Autodesk Fusion 360 part; units mm, degrees
(part 2 of 3)
sketch "Sketch24" plane through (0, 0, 3.2) normal (0, 0, 1) x (-1, 0, 0)
  line L0 (-121.4, -32.3) -> (-121.4, -38.2)
  line L1 (-121.4, -38.2) -> (-118.2, -38.2)
  line L2 (-118.2, -38.2) -> (-118.2, -48.2)
  line L3 (-118.2, -48.2) -> (-121.4, -48.2)
  line L4 (-121.4, -48.2) -> (-121.4, -54.1)
  line L5 (-121.4, -54.1) -> (-118.2, -54.1)
  line L6 (-118.2, -54.1) -> (-118.2, -64.1)
  line L7 (-118.2, -64.1) -> (-121.4, -64.1)
  line L8 (-121.4, -64.1) -> (-121.4, -70)
  line L9 (-121.4, -70) -> (-118.2, -70)
  line L10 (-118.2, -70) -> (-118.2, -80)
  line L11 (-118.2, -80) -> (-121.4, -80)
  line L12 (-121.4, -80) -> (-121.4, -86.4)
  line L13 (-121.4, -86.4) -> (-115, -86.4)
  line L14 (-115, -86.4) -> (-115, -83.2)
  line L15 (-115, -83.2) -> (-105, -83.2)
  line L16 (-105, -83.2) -> (-105, -86.4)
  line L17 (-105, -86.4) -> (-90.35, -86.4)
  line L18 (-90.35, -86.4) -> (-90.35, -83.2)
  line L19 (-90.35, -83.2) -> (-80.35, -83.2)
  line L20 (-80.35, -83.2) -> (-80.35, -86.4)
  line L21 (-80.35, -86.4) -> (-65.7, -86.4)
  line L22 (-65.7, -86.4) -> (-65.7, -83.2)
  line L23 (-65.7, -83.2) -> (-55.7, -83.2)
  line L24 (-55.7, -83.2) -> (-55.7, -86.4)
  line L25 (-55.7, -86.4) -> (-41.05, -86.4)
  line L26 (-41.05, -86.4) -> (-41.05, -83.2)
  line L27 (-41.05, -83.2) -> (-31.05, -83.2)
  line L28 (-31.05, -83.2) -> (-31.05, -86.4)
  line L29 (-31.05, -86.4) -> (-16.4, -86.4)
  line L30 (-16.4, -86.4) -> (-16.4, -83.2)
  line L31 (-16.4, -83.2) -> (-6.4, -83.2)
  line L32 (-6.4, -83.2) -> (-6.4, -86.4)
  line L33 (-6.4, -86.4) -> (0, -86.4)
  line L34 (0, -86.4) -> (0, -80)
  line L35 (0, -80) -> (-3.2, -80)
  line L36 (-3.2, -80) -> (-3.2, -70)
  line L37 (-3.2, -70) -> (0, -70)
  line L38 (0, -70) -> (0, -64.1)
  line L39 (0, -64.1) -> (-3.2, -64.1)
  line L40 (-3.2, -64.1) -> (-3.2, -54.1)
  line L41 (-3.2, -54.1) -> (0, -54.1)
  line L42 (0, -54.1) -> (0, -48.2)
  line L43 (0, -48.2) -> (-3.2, -48.2)
  line L44 (-3.2, -48.2) -> (-3.2, -38.2)
  line L45 (-3.2, -38.2) -> (0, -38.2)
  line L46 (0, -38.2) -> (0, -32.3)
  line L47 (0, -32.3) -> (-3.2, -32.3)
  line L48 (-3.2, -32.3) -> (-3.2, -22.3)
  line L49 (-3.2, -22.3) -> (0, -22.3)
  line L50 (0, -22.3) -> (0, -16.4)
  line L51 (0, -16.4) -> (-3.2, -16.4)
  line L52 (-3.2, -16.4) -> (-3.2, -6.4)
  line L53 (-3.2, -6.4) -> (0, -6.4)
  line L54 (0, -6.4) -> (0, 0)
  line L55 (0, 0) -> (-6.4, 0)
  line L56 (-6.4, 0) -> (-6.4, -3.2)
  line L57 (-6.4, -3.2) -> (-16.4, -3.2)
  line L58 (-16.4, -3.2) -> (-16.4, 0)
  line L59 (-16.4, 0) -> (-31.05, 0)
  line L60 (-31.05, 0) -> (-31.05, -3.2)
  line L61 (-31.05, -3.2) -> (-41.05, -3.2)
  line L62 (-41.05, -3.2) -> (-41.05, 0)
  line L63 (-41.05, 0) -> (-55.7, 0)
  line L64 (-55.7, 0) -> (-55.7, -3.2)
  line L65 (-55.7, -3.2) -> (-65.7, -3.2)
  line L66 (-65.7, -3.2) -> (-65.7, 0)
  line L67 (-65.7, 0) -> (-80.35, 0)
  line L68 (-80.35, 0) -> (-80.35, -3.2)
  line L69 (-80.35, -3.2) -> (-90.35, -3.2)
  line L70 (-90.35, -3.2) -> (-90.35, 0)
  line L71 (-90.35, 0) -> (-105, 0)
  line L72 (-105, 0) -> (-105, -3.2)
  line L73 (-105, -3.2) -> (-115, -3.2)
  line L74 (-115, -3.2) -> (-115, 0)
  line L75 (-115, 0) -> (-121.4, 0)
  line L76 (-121.4, 0) -> (-121.4, -6.4)
  line L77 (-121.4, -6.4) -> (-118.2, -6.4)
  line L78 (-118.2, -6.4) -> (-118.2, -16.4)
  line L79 (-118.2, -16.4) -> (-121.4, -16.4)
  line L80 (-121.4, -16.4) -> (-121.4, -22.3)
  line L81 (-121.4, -22.3) -> (-118.2, -22.3)
  line L82 (-118.2, -22.3) -> (-118.2, -32.3)
  line L83 (-118.2, -32.3) -> (-121.4, -32.3)
  line L84 (-8.2, -83.2) -> (-21.2, -83.2)
  line L85 (-23.2, -81.2) -> (-23.2, -80.2)
  line L86 (-21.2, -78.2) -> (-20.2, -78.2)
  line L87 (-18.2, -76.2) -> (-18.2, -35.2)
  line L88 (-20.2, -33.2) -> (-21.2, -33.2)
  line L89 (-23.2, -31.2) -> (-23.2, -5.2)
  line L90 (-21.2, -3.2) -> (-10.2, -3.2)
  line L91 (-8.2, -5.2) -> (-8.2, -26.2)
  line L92 (-6.2, -28.2) -> (-5.2, -28.2)
  line L93 (-3.2, -30.2) -> (-3.2, -81.2)
  line L94 (-5.2, -83.2) -> (-8.2, -83.2)
  arc A0 (-5.2, -83.2) -> (-3.2, -81.2) centre (-5.2, -81.2) ccw
  arc A1 (-23.2, -81.2) -> (-21.2, -83.2) centre (-21.2, -81.2) ccw
  arc A2 (-21.2, -78.2) -> (-23.2, -80.2) centre (-21.2, -80.2) ccw
  arc A3 (-20.2, -78.2) -> (-18.2, -76.2) centre (-20.2, -76.2) ccw
  arc A4 (-18.2, -35.2) -> (-20.2, -33.2) centre (-20.2, -35.2) ccw
  arc A5 (-23.2, -31.2) -> (-21.2, -33.2) centre (-21.2, -31.2) ccw
  arc A6 (-21.2, -3.2) -> (-23.2, -5.2) centre (-21.2, -5.2) ccw
  arc A7 (-8.2, -5.2) -> (-10.2, -3.2) centre (-10.2, -5.2) ccw
  arc A8 (-8.2, -26.2) -> (-6.2, -28.2) centre (-6.2, -26.2) ccw
  arc A9 (-3.2, -30.2) -> (-5.2, -28.2) centre (-5.2, -30.2) ccw
  line L95 (-23.2, -81.2) -> (-23.2, -70.2)
  line L96 (-25.2, -83.2) -> (-38.7, -83.2)
  line L97 (-40.7, -81.2) -> (-40.7, -80.2)
  line L98 (-42.7, -78.2) -> (-43.7, -78.2)
  line L99 (-45.7, -80.2) -> (-45.7, -81.2)
  line L100 (-47.7, -83.2) -> (-101.2, -83.2)
  line L101 (-25.2, -68.2) -> (-36.2, -68.2)
  line L102 (-38.2, -66.2) -> (-38.2, -65.2)
  line L103 (-40.2, -63.2) -> (-46.2, -63.2)
  line L104 (-48.2, -65.2) -> (-48.2, -66.2)
  line L105 (-50.2, -68.2) -> (-101.2, -68.2)
  line L106 (-103.2, -81.2) -> (-103.2, -70.2)
  arc A10 (-25.2, -83.2) -> (-23.2, -81.2) centre (-25.2, -81.2) ccw
  arc A11 (-23.2, -70.2) -> (-25.2, -68.2) centre (-25.2, -70.2) ccw
  arc A12 (-40.7, -81.2) -> (-38.7, -83.2) centre (-38.7, -81.2) ccw
  arc A13 (-40.7, -80.2) -> (-42.7, -78.2) centre (-42.7, -80.2) ccw
  arc A14 (-47.7, -83.2) -> (-45.7, -81.2) centre (-47.7, -81.2) ccw
  arc A15 (-43.7, -78.2) -> (-45.7, -80.2) centre (-43.7, -80.2) ccw
  arc A16 (-103.2, -81.2) -> (-101.2, -83.2) centre (-101.2, -81.2) ccw
  arc A17 (-101.2, -68.2) -> (-103.2, -70.2) centre (-101.2, -70.2) ccw
  arc A18 (-50.2, -68.2) -> (-48.2, -66.2) centre (-50.2, -66.2) ccw
  arc A19 (-46.2, -63.2) -> (-48.2, -65.2) centre (-46.2, -65.2) ccw
  arc A20 (-38.2, -65.2) -> (-40.2, -63.2) centre (-40.2, -65.2) ccw
  arc A21 (-38.2, -66.2) -> (-36.2, -68.2) centre (-36.2, -66.2) ccw
  line L107 (-18.2, -66.2) -> (-18.2, -55.2)
  line L108 (-20.2, -68.2) -> (-36.2, -68.2)
  line L109 (-38.2, -66.2) -> (-38.2, -65.2)
  line L110 (-40.2, -63.2) -> (-46.2, -63.2)
  line L111 (-48.2, -65.2) -> (-48.2, -66.2)
  line L112 (-50.2, -68.2) -> (-96.2, -68.2)
  line L113 (-98.2, -66.2) -> (-98.2, -55.2)
  arc A22 (-20.2, -68.2) -> (-18.2, -66.2) centre (-20.2, -66.2) ccw
  line L114 (-96.2, -53.2) -> (-55.2, -53.2)
  line L115 (-53.2, -51.2) -> (-53.2, -50.2)
  line L116 (-51.2, -48.2) -> (-35.2, -48.2)
  line L117 (-33.2, -50.2) -> (-33.2, -51.2)
  line L118 (-31.2, -53.2) -> (-20.2, -53.2)
  arc A23 (-38.2, -66.2) -> (-36.2, -68.2) centre (-36.2, -66.2) ccw
  arc A24 (-38.2, -65.2) -> (-40.2, -63.2) centre (-40.2, -65.2) ccw
  arc A25 (-46.2, -63.2) -> (-48.2, -65.2) centre (-46.2, -65.2) ccw
  arc A26 (-50.2, -68.2) -> (-48.2, -66.2) centre (-50.2, -66.2) ccw
  arc A27 (-98.2, -66.2) -> (-96.2, -68.2) centre (-96.2, -66.2) ccw
  arc A28 (-96.2, -53.2) -> (-98.2, -55.2) centre (-96.2, -55.2) ccw
  arc A29 (-55.2, -53.2) -> (-53.2, -51.2) centre (-55.2, -51.2) ccw
  arc A30 (-51.2, -48.2) -> (-53.2, -50.2) centre (-51.2, -50.2) ccw
  arc A31 (-33.2, -50.2) -> (-35.2, -48.2) centre (-35.2, -50.2) ccw
  arc A32 (-33.2, -51.2) -> (-31.2, -53.2) centre (-31.2, -51.2) ccw
  arc A33 (-18.2, -55.2) -> (-20.2, -53.2) centre (-20.2, -55.2) ccw
  line L119 (-18.2, -51.2) -> (-18.2, -38.2)
  line L120 (-20.2, -53.2) -> (-31.2, -53.2)
  line L121 (-33.2, -51.2) -> (-33.2, -50.2)
  line L122 (-35.2, -48.2) -> (-51.2, -48.2)
  line L123 (-53.2, -50.2) -> (-53.2, -51.2)
  line L124 (-55.2, -53.2) -> (-96.2, -53.2)
  line L125 (-98.2, -51.2) -> (-98.2, -40.2)
  line L126 (-96.2, -38.2) -> (-60.2, -38.2)
  line L127 (-58.2, -36.2) -> (-58.2, -35.2)
  line L128 (-56.2, -33.2) -> (-20.2, -33.2)
  line L129 (-18.2, -35.2) -> (-18.2, -38.2)
  arc A34 (-20.2, -53.2) -> (-18.2, -51.2) centre (-20.2, -51.2) ccw
  arc A35 (-33.2, -51.2) -> (-31.2, -53.2) centre (-31.2, -51.2) ccw
  arc A36 (-33.2, -50.2) -> (-35.2, -48.2) centre (-35.2, -50.2) ccw
  arc A37 (-55.2, -53.2) -> (-53.2, -51.2) centre (-55.2, -51.2) ccw
  arc A38 (-51.2, -48.2) -> (-53.2, -50.2) centre (-51.2, -50.2) ccw
  arc A39 (-98.2, -51.2) -> (-96.2, -53.2) centre (-96.2, -51.2) ccw
  arc A40 (-96.2, -38.2) -> (-98.2, -40.2) centre (-96.2, -40.2) ccw
  arc A41 (-60.2, -38.2) -> (-58.2, -36.2) centre (-60.2, -36.2) ccw
  arc A42 (-56.2, -33.2) -> (-58.2, -35.2) centre (-56.2, -35.2) ccw
  line L130 (-23.2, -31.2) -> (-23.2, -20.2)
  line L131 (-23.2, -18.2) -> (-23.2, -5.2)
  arc A43 (-18.2, -35.2) -> (-20.2, -33.2) centre (-20.2, -35.2) ccw
  line L132 (-25.2, -33.2) -> (-56.2, -33.2)
  line L133 (-58.2, -35.2) -> (-58.2, -36.2)
  line L134 (-60.2, -38.2) -> (-101.2, -38.2)
  line L135 (-103.2, -36.2) -> (-103.2, -20.2)
  line L136 (-101.2, -18.2) -> (-100.2, -18.2)
  line L137 (-98.2, -20.2) -> (-98.2, -21.2)
  line L138 (-96.2, -23.2) -> (-90.2, -23.2)
  line L139 (-88.2, -21.2) -> (-88.2, -20.2)
  line L140 (-86.2, -18.2) -> (-25.2, -18.2)
  arc A44 (-25.2, -33.2) -> (-23.2, -31.2) centre (-25.2, -31.2) ccw
  arc A45 (-56.2, -33.2) -> (-58.2, -35.2) centre (-56.2, -35.2) ccw
  arc A46 (-60.2, -38.2) -> (-58.2, -36.2) centre (-60.2, -36.2) ccw
  arc A47 (-103.2, -36.2) -> (-101.2, -38.2) centre (-101.2, -36.2) ccw
  arc A48 (-101.2, -18.2) -> (-103.2, -20.2) centre (-101.2, -20.2) ccw
  arc A49 (-98.2, -20.2) -> (-100.2, -18.2) centre (-100.2, -20.2) ccw
  arc A50 (-98.2, -21.2) -> (-96.2, -23.2) centre (-96.2, -21.2) ccw
  arc A51 (-90.2, -23.2) -> (-88.2, -21.2) centre (-90.2, -21.2) ccw
  arc A52 (-86.2, -18.2) -> (-88.2, -20.2) centre (-86.2, -20.2) ccw
  arc A53 (-23.2, -20.2) -> (-25.2, -18.2) centre (-25.2, -20.2) ccw
  line L141 (-23.2, -16.2) -> (-23.2, -3.2)
  line L142 (-25.2, -18.2) -> (-86.2, -18.2)
  line L143 (-88.2, -20.2) -> (-88.2, -21.2)
  line L144 (-90.2, -23.2) -> (-96.2, -23.2)
  line L145 (-98.2, -21.2) -> (-98.2, -20.2)
  line L146 (-100.2, -18.2) -> (-101.2, -18.2)
  line L147 (-103.2, -16.2) -> (-103.2, -5.2)
  line L148 (-101.2, -3.2) -> (-97.7, -3.2)
  line L149 (-95.7, -5.2) -> (-95.7, -6.2)
  line L150 (-93.7, -8.2) -> (-92.7, -8.2)
  line L151 (-90.7, -6.2) -> (-90.7, -5.2)
  line L152 (-88.7, -3.2) -> (-25.2, -3.2)
  arc A54 (-23.2, -5.2) -> (-25.2, -3.2) centre (-25.2, -5.2) ccw
  arc A55 (-25.2, -18.2) -> (-23.2, -16.2) centre (-25.2, -16.2) ccw
  arc A56 (-86.2, -18.2) -> (-88.2, -20.2) centre (-86.2, -20.2) ccw
  arc A57 (-90.2, -23.2) -> (-88.2, -21.2) centre (-90.2, -21.2) ccw
  arc A58 (-98.2, -21.2) -> (-96.2, -23.2) centre (-96.2, -21.2) ccw
  arc A59 (-98.2, -20.2) -> (-100.2, -18.2) centre (-100.2, -20.2) ccw
  arc A60 (-103.2, -16.2) -> (-101.2, -18.2) centre (-101.2, -16.2) ccw
  arc A61 (-101.2, -3.2) -> (-103.2, -5.2) centre (-101.2, -5.2) ccw
  arc A62 (-95.7, -5.2) -> (-97.7, -3.2) centre (-97.7, -5.2) ccw
  arc A63 (-95.7, -6.2) -> (-93.7, -8.2) centre (-93.7, -6.2) ccw
  arc A64 (-92.7, -8.2) -> (-90.7, -6.2) centre (-92.7, -6.2) ccw
  arc A65 (-88.7, -3.2) -> (-90.7, -5.2) centre (-88.7, -5.2) ccw
  line L153 (-116.2, -3.2) -> (-105.2, -3.2)
  line L154 (-103.2, -5.2) -> (-103.2, -36.2)
  line L155 (-101.2, -38.2) -> (-100.2, -38.2)
  line L156 (-98.2, -40.2) -> (-98.2, -66.2)
  line L157 (-100.2, -68.2) -> (-101.2, -68.2)
  line L158 (-103.2, -70.2) -> (-103.2, -81.2)
  line L159 (-105.2, -83.2) -> (-116.2, -83.2)
  line L160 (-118.2, -81.2) -> (-118.2, -62.7)
  line L161 (-116.2, -60.7) -> (-115.2, -60.7)
  line L162 (-113.2, -58.7) -> (-113.2, -47.7)
  line L163 (-115.2, -45.7) -> (-116.2, -45.7)
  line L164 (-118.2, -43.7) -> (-118.2, -5.2)
  arc A66 (-103.2, -5.2) -> (-105.2, -3.2) centre (-105.2, -5.2) ccw
  arc A67 (-116.2, -3.2) -> (-118.2, -5.2) centre (-116.2, -5.2) ccw
  arc A68 (-118.2, -43.7) -> (-116.2, -45.7) centre (-116.2, -43.7) ccw
  arc A69 (-113.2, -47.7) -> (-115.2, -45.7) centre (-115.2, -47.7) ccw
  arc A70 (-115.2, -60.7) -> (-113.2, -58.7) centre (-115.2, -58.7) ccw
  arc A71 (-116.2, -60.7) -> (-118.2, -62.7) centre (-116.2, -62.7) ccw
  arc A72 (-118.2, -81.2) -> (-116.2, -83.2) centre (-116.2, -81.2) ccw
  arc A73 (-105.2, -83.2) -> (-103.2, -81.2) centre (-105.2, -81.2) ccw
  arc A74 (-101.2, -68.2) -> (-103.2, -70.2) centre (-101.2, -70.2) ccw
  arc A75 (-100.2, -68.2) -> (-98.2, -66.2) centre (-100.2, -66.2) ccw
  arc A76 (-98.2, -40.2) -> (-100.2, -38.2) centre (-100.2, -40.2) ccw
  arc A77 (-103.2, -36.2) -> (-101.2, -38.2) centre (-101.2, -36.2) ccw
  point P0 (-23.2, -83.2)
  point P1 (-3.2, -83.2)
  point P2 (-23.2, -78.2)
  point P3 (-18.2, -78.2)
  point P4 (-18.2, -33.2)
  point P5 (-23.2, -33.2)
  point P6 (-23.2, -3.2)
  point P7 (-8.2, -3.2)
  point P8 (-8.2, -28.2)
  point P9 (-3.2, -28.2)
  point P10 (-23.2, -83.2)
  point P11 (-23.2, -68.2)
  point P12 (-40.7, -83.2)
  point P13 (-40.7, -78.2)
  point P14 (-45.7, -78.2)
  point P15 (-45.7, -83.2)
  point P16 (-103.2, -83.2)
  point P17 (-38.2, -68.2)
  point P18 (-38.2, -63.2)
  point P19 (-48.2, -63.2)
  point P20 (-48.2, -68.2)
  point P21 (-103.2, -68.2)
  point P22 (-18.2, -68.2)
  point P23 (-18.2, -53.2)
  point P24 (-38.2, -68.2)
  point P25 (-38.2, -63.2)
  point P26 (-38.2, -63.2)
  point P27 (-48.2, -63.2)
  point P28 (-48.2, -68.2)
  point P29 (-48.2, -68.2)
  point P30 (-98.2, -68.2)
  point P31 (-98.2, -53.2)
  point P32 (-53.2, -53.2)
  point P33 (-53.2, -48.2)
  point P34 (-33.2, -48.2)
  point P35 (-33.2, -53.2)
  point P36 (-18.2, -53.2)
  point P37 (-33.2, -53.2)
  point P38 (-33.2, -48.2)
  point P39 (-33.2, -48.2)
  point P40 (-53.2, -48.2)
  point P41 (-53.2, -48.2)
  point P42 (-53.2, -53.2)
  point P43 (-53.2, -53.2)
  point P44 (-98.2, -53.2)
  point P45 (-98.2, -38.2)
  point P46 (-58.2, -38.2)
  point P47 (-58.2, -33.2)
  point P48 (-18.2, -33.2)
  point P49 (-23.2, -33.2)
  point P50 (-23.2, -3.2)
  point P51 (-23.2, -33.2)
  point P52 (-58.2, -33.2)
  point P53 (-58.2, -38.2)
  point P54 (-58.2, -38.2)
  point P55 (-103.2, -38.2)
  point P56 (-103.2, -18.2)
  point P57 (-98.2, -18.2)
  point P58 (-98.2, -23.2)
  point P59 (-88.2, -23.2)
  point P60 (-88.2, -18.2)
  point P61 (-23.2, -18.2)
  point P62 (-23.2, -18.2)
  point P63 (-88.2, -18.2)
  point P64 (-88.2, -18.2)
  point P65 (-88.2, -23.2)
  point P66 (-98.2, -23.2)
  point P67 (-98.2, -18.2)
  point P68 (-103.2, -18.2)
  point P69 (-103.2, -18.2)
  point P70 (-103.2, -3.2)
  point P71 (-95.7, -3.2)
  point P72 (-95.7, -8.2)
  point P73 (-90.7, -8.2)
  point P74 (-90.7, -3.2)
  point P75 (-118.2, -3.2)
  point P76 (-103.2, -3.2)
  point P77 (-103.2, -38.2)
  point P78 (-103.2, -38.2)
  point P79 (-98.2, -38.2)
  point P80 (-98.2, -38.2)
  point P81 (-98.2, -68.2)
  point P82 (-98.2, -68.2)
  point P83 (-103.2, -68.2)
  point P84 (-103.2, -68.2)
  point P85 (-103.2, -83.2)
  point P86 (-103.2, -83.2)
  point P87 (-118.2, -83.2)
  point P88 (-118.2, -60.7)
  point P89 (-113.2, -60.7)
  point P90 (-113.2, -45.7)
  point P91 (-118.2, -45.7)
  point P92 (-118.2, -3.2)
  dimension "d178" = 15
  dimension "d179" = 5
  dimension "d180" = 5
  dimension "d181" = 5
  dimension "d182" = 45
  dimension "d183" = 5
  dimension "d185" = 15
  dimension "d186" = 25
  dimension "d187" = 5
  dimension "d188" = 2
  dimension "d189" = 8.2
  dimension "d190" = 2
  dimension "d191" = 2
  dimension "d192" = 2
  dimension "d193" = 2
  dimension "d194" = 2
  dimension "d195" = 2
  dimension "d196" = 2
  dimension "d197" = 2
  dimension "d198" = 2
  dimension "d202" = 30
  dimension "d203" = 80
  dimension "d204" = 15
  dimension "d205" = 23.2
  dimension "d206" = 83.2
  dimension "d208" = 17.5
  dimension "d209" = 5
  dimension "d210" = 5
  dimension "d211" = 5
  dimension "d212" = 57.5
  dimension "d213" = 15
  dimension "d214" = 5
  dimension "d215" = 10
  dimension "d216" = 5
  dimension "d218" = 55
  dimension "d219" = 2
  dimension "d220" = 2
  dimension "d221" = 2
  dimension "d222" = 2
  dimension "d223" = 2
  dimension "d224" = 2
  dimension "d225" = 2
  dimension "d226" = 2
  dimension "d227" = 2
  dimension "d228" = 2
  dimension "d229" = 2
  dimension "d230" = 2
  dimension "d231" = 15
  dimension "d232" = 18.2
  dimension "d233" = 68.2
  dimension "d234" = 20
  dimension "d235" = 5
  dimension "d237" = 10
  dimension "d238" = 5
  dimension "d239" = 50
  dimension "d240" = 15
  dimension "d241" = 2
  dimension "d242" = 5
  dimension "d243" = 5
  dimension "d244" = 20
  dimension "d245" = 5
  dimension "d246" = 2
  dimension "d247" = 2
  dimension "d248" = 2
  dimension "d249" = 2
  dimension "d250" = 2
  dimension "d251" = 2
  dimension "d252" = 2
  dimension "d253" = 2
  dimension "d254" = 2
  dimension "d255" = 2
  dimension "d256" = 2
  dimension "d257" = 15
  dimension "d258" = 18.2
  dimension "d259" = 53.2
  dimension "d260" = 15
  dimension "d261" = 5
  dimension "d262" = 20
  dimension "d263" = 5
  dimension "d264" = 45
  dimension "d265" = 15
  dimension "d266" = 40
  dimension "d267" = 5
  dimension "d268" = 40
  dimension "d269" = 2
  dimension "d270" = 2
  dimension "d271" = 2
  dimension "d272" = 2
  dimension "d273" = 2
  dimension "d274" = 2
  dimension "d275" = 2
  dimension "d276" = 2
  dimension "d277" = 2
  dimension "d278" = 15
  dimension "d279" = 23.2
  dimension "d280" = 33.2
  dimension "d281" = 2
  dimension "d282" = 35
  dimension "d283" = 5
  dimension "d284" = 45
  dimension "d285" = 20
  dimension "d286" = 5
  dimension "d287" = 5
  dimension "d288" = 10
  dimension "d289" = 5
  dimension "d290" = 65
  dimension "d291" = 15
  dimension "d292" = 40
  dimension "d293" = 2
  dimension "d294" = 2
  dimension "d295" = 2
  dimension "d296" = 2
  dimension "d297" = 2
  dimension "d298" = 2
  dimension "d299" = 2
  dimension "d300" = 2
  dimension "d301" = 2
  dimension "d302" = 2
  dimension "d303" = 15
  dimension "d304" = 3.2
  dimension "d305" = 23.2
  dimension "d306" = 65
  dimension "d307" = 5
  dimension "d308" = 10
  dimension "d309" = 5
  dimension "d310" = 5
  dimension "d311" = 15
  dimension "d312" = 7.5
  dimension "d313" = 5
  dimension "d314" = 5
  dimension "d315" = 5
  dimension "d316" = 2
  dimension "d317" = 2
  dimension "d318" = 2
  dimension "d319" = 2
  dimension "d320" = 2
  dimension "d321" = 2
  dimension "d322" = 2
  dimension "d323" = 2
  dimension "d324" = 2
  dimension "d325" = 2
  dimension "d326" = 2
  dimension "d327" = 2
  dimension "d328" = 15
  dimension "d330" = 15
  dimension "d331" = 3.2
  dimension "d332" = 103.2
  dimension "d333" = 35
  dimension "d334" = 5
  dimension "d335" = 30
  dimension "d336" = 5
  dimension "d337" = 15
  dimension "d338" = 15
  dimension "d339" = 22.5
  dimension "d340" = 5
  dimension "d341" = 15
  dimension "d342" = 5
  dimension "d343" = 42.5
  dimension "d344" = 2
  dimension "d345" = 2
  dimension "d346" = 2
  dimension "d347" = 2
  dimension "d348" = 2
  dimension "d349" = 2
  dimension "d350" = 2
  dimension "d351" = 2
  dimension "d352" = 2
  dimension "d353" = 2
  dimension "d354" = 2
  dimension "d355" = 2
  constraint perpendicular L32 L84
  constraint perpendicular L84 L85
  constraint perpendicular L85 L86
  constraint perpendicular L86 L87
  constraint perpendicular L87 L88
  constraint perpendicular L88 L89
  constraint perpendicular L89 L90
  constraint perpendicular L57 L91
  constraint perpendicular L91 L92
  constraint perpendicular L35 L93
  constraint perpendicular L32 L94
  constraint tangent L93 A0
  constraint tangent L94 A0
  constraint coincident P10 L84
  constraint coincident P10 L85
  constraint tangent L84 A1
  constraint tangent L85 A1
  constraint coincident P2 L85
  constraint coincident P2 L86
  constraint tangent L85 A2
  constraint tangent L86 A2
  constraint coincident P3 L86
  constraint coincident P3 L87
  constraint tangent L86 A3
  constraint tangent L87 A3
  constraint coincident P48 L88
  constraint tangent L87 A4
  constraint tangent L88 A4
  constraint coincident P51 L88
  constraint coincident P51 L89
  constraint tangent L88 A5
  constraint tangent L89 A5
  constraint coincident P50 L89
  constraint coincident P50 L90
  constraint tangent L89 A6
  constraint tangent L90 A6
  constraint coincident P7 L90
  constraint coincident P7 L91
  constraint tangent L90 A7
  constraint tangent L91 A7
  constraint coincident P8 L91
  constraint coincident P8 L92
  constraint tangent L91 A8
  constraint tangent L92 A8
  constraint coincident P9 L92
  constraint coincident P9 L93
  constraint tangent L92 A9
  constraint tangent L93 A9
  constraint vertical L95
  constraint perpendicular L26 L96
  constraint perpendicular L27 L97
  constraint perpendicular L97 L98
  constraint perpendicular L98 L99
  constraint perpendicular L20 L100
  constraint perpendicular L95 L101
  constraint perpendicular L101 L102
  constraint perpendicular L102 L103
  constraint perpendicular L103 L104
  constraint perpendicular L104 L105
  constraint coincident P10 L95
  constraint coincident P10 L96
  constraint tangent L95 A10
  constraint tangent L96 A10
  constraint coincident P11 L95
  constraint coincident P11 L101
  constraint tangent L95 A11
  constraint tangent L101 A11
  constraint coincident P12 L96
  constraint coincident P12 L97
  constraint tangent L96 A12
  constraint tangent L97 A12
  constraint coincident P13 L97
  constraint coincident P13 L98
  constraint tangent L97 A13
  constraint tangent L98 A13
  constraint coincident P15 L99
  constraint coincident P15 L100
  constraint tangent L99 A14
  constraint tangent L100 A14
  constraint coincident P14 L98
  constraint coincident P14 L99
  constraint tangent L98 A15
  constraint tangent L99 A15
  constraint coincident P86 L100
  constraint coincident P86 L106
  constraint tangent L100 A16
  constraint tangent L106 A16
  constraint coincident P84 L105
  constraint coincident P84 L106
  constraint tangent L105 A17
  constraint tangent L106 A17
  constraint coincident P29 L104
  constraint coincident P29 L105
  constraint tangent L104 A18
  constraint tangent L105 A18
  constraint coincident P27 L103
  constraint coincident P27 L104
  constraint tangent L103 A19
  constraint tangent L104 A19
  constraint coincident P26 L102
  constraint coincident P26 L103
  constraint tangent L102 A20
  constraint tangent L103 A20
  constraint coincident P24 L101
  constraint coincident P24 L102
  constraint tangent L101 A21
  constraint tangent L102 A21
  constraint parallel L87 L107
  constraint perpendicular L107 L108
  constraint perpendicular L108 L109
  constraint coincident P26 P25
  constraint perpendicular L109 L110
  constraint vertical L111
  constraint coincident P29 P28
  constraint perpendicular L111 L112
  constraint perpendicular L105 L113
  constraint coincident P22 L107
  constraint coincident P22 L108
  constraint tangent L107 A22
  constraint tangent L108 A22
  constraint perpendicular L113 L114
  constraint perpendicular L114 L115
  constraint perpendicular L115 L116
  constraint perpendicular L116 L117
  constraint coincident P24 L109
  constraint coincident P24 L108
  constraint tangent L109 A23
  constraint tangent L108 A23
  constraint coincident P26 L109
  constraint coincident P26 L110
  constraint tangent L109 A24
  constraint tangent L110 A24
  constraint coincident P27 L110
  constraint coincident P27 L111
  constraint tangent L110 A25
  constraint tangent L111 A25
  constraint coincident P29 L111
  constraint coincident P29 L112
  constraint tangent L111 A26
  constraint tangent L112 A26
  constraint coincident P82 L112
  constraint coincident P82 L113
  constraint tangent L112 A27
  constraint tangent L113 A27
  constraint coincident P44 L113
  constraint coincident P44 L114
  constraint tangent L113 A28
  constraint tangent L114 A28
  constraint coincident P43 L114
  constraint coincident P43 L115
  constraint tangent L114 A29
  constraint tangent L115 A29
  constraint coincident P41 L115
  constraint coincident P41 L116
  constraint tangent L115 A30
  constraint tangent L116 A30
  constraint coincident P39 L116
  constraint coincident P39 L117
  constraint tangent L116 A31
  constraint tangent L117 A31
  constraint coincident P37 L117
  constraint coincident P37 L118
  constraint tangent L117 A32
  constraint tangent L118 A32
  constraint coincident P36 L107
  constraint coincident P36 L118
  constraint tangent L107 A33
  constraint tangent L118 A33
  constraint vertical L119
  constraint perpendicular L87 L120
  constraint perpendicular L120 L121
  constraint coincident P39 P38
  constraint perpendicular L121 L122
  constraint coincident P41 P40
  constraint perpendicular L122 L123
  constraint coincident P43 P42
  constraint perpendicular L113 L124
  constraint perpendicular L124 L125
  constraint perpendicular L125 L126
  constraint perpendicular L126 L127
  constraint perpendicular L127 L128
  constraint coincident P36 L120
  constraint coincident P36 L119
  constraint tangent L120 A34
  constraint tangent L119 A34
  constraint coincident P37 L121
  constraint coincident P37 L120
  constraint tangent L121 A35
  constraint tangent L120 A35
  constraint coincident P39 L121
  constraint coincident P39 L122
  constraint tangent L121 A36
  constraint tangent L122 A36
  constraint coincident P43 L124
  constraint coincident P43 L123
  constraint tangent L124 A37
  constraint tangent L123 A37
  constraint coincident P41 L123
  constraint coincident P41 L122
  constraint tangent L123 A38
  constraint tangent L122 A38
  constraint coincident P44 L124
  constraint coincident P44 L125
  constraint tangent L124 A39
  constraint tangent L125 A39
  constraint coincident P80 L125
  constraint coincident P80 L126
  constraint tangent L125 A40
  constraint tangent L126 A40
  constraint coincident P54 L126
  constraint coincident P54 L127
  constraint tangent L126 A41
  constraint tangent L127 A41
  constraint coincident P52 L127
  constraint coincident P52 L128
  constraint tangent L127 A42
  constraint tangent L128 A42
  constraint perpendicular L118 L130
  constraint perpendicular L118 L131
  constraint coincident P48 L128
  constraint tangent L129 A43
  constraint tangent L128 A43
  constraint coincident P51 P49
  constraint parallel L128 L132
  constraint perpendicular L132 L133
  constraint coincident P54 P53
  constraint perpendicular L133 L134
  constraint perpendicular L134 L135
  constraint perpendicular L135 L136
  constraint perpendicular L136 L137
  constraint perpendicular L137 L138
  constraint perpendicular L138 L139
  constraint perpendicular L89 L140
  constraint coincident P51 L130
  constraint coincident P51 L132
  constraint tangent L130 A44
  constraint tangent L132 A44
  constraint coincident P52 L132
  constraint coincident P52 L133
  constraint tangent L132 A45
  constraint tangent L133 A45
  constraint coincident P54 L134
  constraint coincident P54 L133
  constraint tangent L134 A46
  constraint tangent L133 A46
  constraint coincident P78 L134
  constraint coincident P78 L135
  constraint tangent L134 A47
  constraint tangent L135 A47
  constraint coincident P69 L135
  constraint coincident P69 L136
  constraint tangent L135 A48
  constraint tangent L136 A48
  constraint coincident P67 L136
  constraint coincident P67 L137
  constraint tangent L136 A49
  constraint tangent L137 A49
  constraint coincident P66 L137
  constraint coincident P66 L138
  constraint tangent L137 A50
  constraint tangent L138 A50
  constraint coincident P65 L138
  constraint coincident P65 L139
  constraint tangent L138 A51
  constraint tangent L139 A51
  constraint coincident P64 L139
  constraint coincident P64 L140
  constraint tangent L139 A52
  constraint tangent L140 A52
  constraint coincident P62 L140
  constraint coincident P62 L130
  constraint tangent L140 A53
  constraint tangent L130 A53
  constraint vertical L141
  constraint perpendicular L89 L142
  constraint coincident P64 P63
  constraint perpendicular L142 L143
  constraint perpendicular L143 L144
  constraint perpendicular L144 L145
  constraint perpendicular L145 L146
  constraint coincident P69 P68
  constraint perpendicular L146 L147
  constraint perpendicular L147 L148
  constraint perpendicular L148 L149
  constraint perpendicular L149 L150
  constraint perpendicular L69 L151
  constraint coincident P50 L131
  constraint tangent L131 A54
  constraint tangent L152 A54
  constraint coincident P62 L141
  constraint coincident P62 L142
  constraint tangent L141 A55
  constraint tangent L142 A55
  constraint coincident P64 L142
  constraint coincident P64 L143
  constraint tangent L142 A56
  constraint tangent L143 A56
  constraint coincident P65 L144
  constraint coincident P65 L143
  constraint tangent L144 A57
  constraint tangent L143 A57
  constraint coincident P66 L144
  constraint coincident P66 L145
  constraint tangent L144 A58
  constraint tangent L145 A58
  constraint coincident P67 L145
  constraint coincident P67 L146
  constraint tangent L145 A59
  constraint tangent L146 A59
  constraint coincident P69 L147
  constraint coincident P69 L146
  constraint tangent L147 A60
  constraint tangent L146 A60
  constraint coincident P76 L147
  constraint coincident P76 L148
  constraint tangent L147 A61
  constraint tangent L148 A61
  constraint coincident P71 L148
  constraint coincident P71 L149
  constraint tangent L148 A62
  constraint tangent L149 A62
  constraint coincident P72 L149
  constraint coincident P72 L150
  constraint tangent L149 A63
  constraint tangent L150 A63
  constraint coincident P73 L150
  constraint coincident P73 L151
  constraint tangent L150 A64
  constraint tangent L151 A64
  constraint coincident P74 L151
  constraint coincident P74 L152
  constraint tangent L151 A65
  constraint tangent L152 A65
  constraint parallel L73 L153
  constraint perpendicular L153 L154
  constraint coincident P78 P77
  constraint perpendicular L154 L155
  constraint coincident P80 P79
  constraint perpendicular L105 L156
  constraint coincident P82 P81
  constraint perpendicular L156 L157
  constraint coincident P84 P83
  constraint perpendicular L157 L158
  constraint coincident P86 P85
  constraint perpendicular L158 L159
  constraint perpendicular L159 L160
  constraint perpendicular L160 L161
  constraint perpendicular L161 L162
  constraint perpendicular L2 L163
  constraint perpendicular L79 L164
  constraint coincident P76 L153
  constraint coincident P76 L154
  constraint tangent L153 A66
  constraint tangent L154 A66
  constraint coincident P92 L153
  constraint coincident P92 L164
  constraint tangent L153 A67
  constraint tangent L164 A67
  constraint coincident P91 L163
  constraint coincident P91 L164
  constraint tangent L163 A68
  constraint tangent L164 A68
  constraint coincident P90 L162
  constraint coincident P90 L163
  constraint tangent L162 A69
  constraint tangent L163 A69
  constraint coincident P89 L161
  constraint coincident P89 L162
  constraint tangent L161 A70
  constraint tangent L162 A70
  constraint coincident P88 L160
  constraint coincident P88 L161
  constraint tangent L160 A71
  constraint tangent L161 A71
  constraint coincident P87 L159
  constraint coincident P87 L160
  constraint tangent L159 A72
  constraint tangent L160 A72
  constraint coincident P86 L158
  constraint coincident P86 L159
  constraint tangent L158 A73
  constraint tangent L159 A73
  constraint coincident P84 L157
  constraint coincident P84 L158
  constraint tangent L157 A74
  constraint tangent L158 A74
  constraint coincident P82 L156
  constraint coincident P82 L157
  constraint tangent L156 A75
  constraint tangent L157 A75
  constraint coincident P80 L156
  constraint coincident P80 L155
  constraint tangent L156 A76
  constraint tangent L155 A76
  constraint coincident P78 L155
  constraint coincident P78 L154
  constraint tangent L155 A77
  constraint tangent L154 A77
  measures "d178" distance of L84.start P10
  measures "d179" distance of L84.start P1
  measures "d180" distance of P10 P2
  measures "d181" distance of P2 P3
  measures "d182" distance of P3 P48
  measures "d183" distance of P48 P51
  measures "d185" distance of P50 P7
  measures "d186" distance of P7 P8
  measures "d187" distance of P8 P9
  measures "d188" radius of A0
  measures "d189" horizontal distance of L54.end P7
  measures "d190" radius of A1
  measures "d191" radius of A2
  measures "d192" radius of A3
  measures "d193" radius of A4
  measures "d194" radius of A5
  measures "d195" radius of A6
  measures "d196" radius of A7
  measures "d197" radius of A8
  measures "d198" radius of A9
  measures "d202" distance of L88 L90
  measures "d203" distance of L57.end L84
  measures "d204" distance of P10 P11
  measures "d205" horizontal distance of L54.end P10
  measures "d206" vertical distance of L54.end P10
  measures "d208" distance of P10 P12
  measures "d209" distance of P12 P13
  measures "d210" distance of P13 P14
  measures "d211" distance of P14 P15
  measures "d212" distance of P15 P86
  measures "d213" distance of P11 P24
  measures "d214" distance of P24 P26
  measures "d215" distance of P26 P27
  measures "d216" distance of P27 P29
  measures "d218" distance of P29 P84
  measures "d219" radius of A10
  measures "d220" radius of A11
  measures "d221" radius of A12
  measures "d222" radius of A13
  measures "d223" radius of A14
  measures "d224" radius of A15
  measures "d225" radius of A16
  measures "d226" radius of A17
  measures "d227" radius of A18
  measures "d228" radius of A19
  measures "d229" radius of A20
  measures "d230" radius of A21
  measures "d231" distance of P22 P36
  measures "d232" distance of L54.end L107
  measures "d233" vertical distance of L54.end P22
  measures "d234" distance of P22 P24
  measures "d235" distance of P24 P26
  measures "d237" distance of P26 P27
  measures "d238" distance of P27 P29
  measures "d239" distance of P29 P82
  measures "d240" distance of P82 P44
  measures "d241" radius of A22
  measures "d242" horizontal distance of P27 P43
  measures "d243" distance of P43 P41
  measures "d244" distance of P41 P39
  measures "d245" distance of P39 P37
  measures "d246" radius of A23
  measures "d247" radius of A24
  measures "d248" radius of A25
  measures "d249" radius of A26
  measures "d250" radius of A27
  measures "d251" radius of A28
  measures "d252" radius of A29
  measures "d253" radius of A30
  measures "d254" radius of A31
  measures "d255" radius of A32
  measures "d256" radius of A33
  measures "d257" distance of P36 L119.end
  measures "d258" horizontal distance of L54.end P36
  measures "d259" vertical distance of L54.end P36
  measures "d260" distance of P36 P37
  measures "d261" distance of P37 P39
  measures "d262" distance of P39 P41
  measures "d263" distance of P41 P43
  measures "d264" distance of P43 P44
  measures "d265" distance of P44 P80
  measures "d266" distance of P80 P54
  measures "d267" distance of P54 P52
  measures "d268" distance of P52 P48
  measures "d269" radius of A34
  measures "d270" radius of A35
  measures "d271" radius of A36
  measures "d272" radius of A37
  measures "d273" radius of A38
  measures "d274" radius of A39
  measures "d275" radius of A40
  measures "d276" radius of A41
  measures "d277" radius of A42
  measures "d278" distance of P62 P50
  measures "d279" horizontal distance of L54.end P51
  measures "d280" vertical distance of L54.end P51
  measures "d281" radius of A43
  measures "d282" distance of P51 P52
  measures "d283" distance of P52 P54
  measures "d284" distance of P54 P78
  measures "d285" distance of P78 P69
  measures "d286" distance of P69 P67
  measures "d287" distance of P67 P66
  measures "d288" distance of P66 P65
  measures "d289" distance of P65 P64
  measures "d290" distance of P64 P62
  measures "d291" distance of P51 P62
  measures "d292" distance of P52 L129
  measures "d293" radius of A44
  measures "d294" radius of A45
  measures "d295" radius of A46
  measures "d296" radius of A47
  measures "d297" radius of A48
  measures "d298" radius of A49
  measures "d299" radius of A50
  measures "d300" radius of A51
  measures "d301" radius of A52
  measures "d302" radius of A53
  measures "d303" distance of P62 P50
  measures "d304" vertical distance of L54.end P50
  measures "d305" distance of L54.end L141
  measures "d306" distance of P62 P64
  measures "d307" distance of P64 P65
  measures "d308" distance of P65 P66
  measures "d309" distance of P66 P67
  measures "d310" distance of P67 P69
  measures "d311" distance of P69 P76
  measures "d312" distance of P76 P71
  measures "d313" distance of P71 P72
  measures "d314" distance of P72 P73
  measures "d315" distance of P73 P74
  measures "d316" radius of A54
  measures "d317" radius of A55
  measures "d318" radius of A56
  measures "d319" radius of A57
  measures "d320" radius of A58
  measures "d321" radius of A59
  measures "d322" radius of A60
  measures "d323" radius of A61
  measures "d324" radius of A62
  measures "d325" radius of A63
  measures "d326" radius of A64
  measures "d327" radius of A65
  measures "d328" distance of L142 L152
  measures "d330" distance of P92 P76
  measures "d331" vertical distance of L54.end P92
  measures "d332" horizontal distance of L54.end P76
  measures "d333" distance of P76 P78
  measures "d334" distance of P78 P80
  measures "d335" distance of P80 P82
  measures "d336" distance of P82 P84
  measures "d337" distance of P84 P86
  measures "d338" distance of P86 P87
  measures "d339" distance of P87 P88
  measures "d340" distance of P88 P89
  measures "d341" distance of P89 P90
  measures "d342" distance of P90 P91
  measures "d343" distance of P91 P92
  measures "d344" radius of A66
  measures "d345" radius of A67
  measures "d346" radius of A68
  measures "d347" radius of A69
  measures "d348" radius of A70
  measures "d349" radius of A71
  measures "d350" radius of A72
  measures "d351" radius of A73
  measures "d352" radius of A74
  measures "d353" radius of A75
  measures "d354" radius of A76
  measures "d355" radius of A77
extrude "Extrude27" add sketch "Sketch24" along normal blind 2 separate body contours L31 L36 L40 L44 L48 L57 L84 L85 L86 L87 L88 L89 L90 L91 L92 L93 L94 A0 A1 A2 A3 A4 A5 A6 A7 A8 A9 L95 L107 L119 L128 L129 L130 L131 A43 L141 makes body 22
extrude "Extrude28" add sketch "Sketch24" along normal blind 2 separate body contours L19 L23 L27 L85 L95 L96 L97 L98 L99 L100 L101 L102 L103 L104 L105 L106 A10 A11 A12 A13 A14 A15 A16 A17 A18 A19 A20 A21 L108 L109 L110 L111 L112 A23 A24 A25 A26 L157 L158 A74 makes body 23
extrude "Extrude29" add sketch "Sketch24" along normal blind 2 separate body contours L87 L101 L102 L103 L104 L105 A18 A19 A20 A21 L107 L108 L109 L110 L111 L112 L113 A22 L114 L115 L116 L117 L118 A23 A24 A25 A26 A27 A28 A29 A30 A31 A32 A33 L120 L121 L122 L123 L124 A35 A36 A37 A38 L156 makes body 24
extrude "Extrude30" add sketch "Sketch24" along normal blind 2 separate body contours L87 L88 A4 L114 L115 L116 L117 L118 A29 A30 A31 A32 L119 L120 L121 L122 L123 L124 L125 L126 L127 L128 L129 A34 A35 A36 A37 A38 A39 A40 A41 A42 A43 L132 L133 L134 A45 A46 L156 makes body 25
extrude "Extrude31" add sketch "Sketch24" along normal blind 2 separate body contours L89 L126 L127 L128 A41 A42 L130 L132 L133 L134 L135 L136 L137 L138 L139 L140 A44 A45 A46 A47 A48 A49 A50 A51 A52 A53 L142 L143 L144 L145 L146 A56 A57 A58 A59 L154 L155 A77 makes body 26
extrude "Extrude32" add sketch "Sketch24" along normal blind 2 separate body contours L61 L65 L69 L89 L131 L136 L137 L138 L139 L140 A49 A50 A51 A52 L141 L142 L143 L144 L145 L146 L147 L148 L149 L150 L151 L152 A54 A55 A56 A57 A58 A59 A60 A61 A62 A63 A64 A65 L154 makes body 27
extrude "Extrude33" add sketch "Sketch24" along normal blind 2 separate body contours L2 L6 L10 L15 L73 L78 L82 L105 L106 A17 L113 L125 L134 L135 A47 L147 L153 L154 L155 L156 L157 L158 L159 L160 L161 L162 L163 L164 A66 A67 A68 A69 A70 A71 A72 A73 A74 A75 A76 A77 makes body 28
copy_body "Body->Comp1" bodies 1 removing the originals makes body 29 in component "Component"
copy_body "Body->Comp2" bodies 2 removing the originals makes body 30 in component "Component'"
copy_body "Body->Comp3" bodies 7 removing the originals makes body 31 in component "Component''"
copy_body "Body->Comp4" bodies 12 removing the originals makes body 32 in component "Component'''"
copy_body "Body->Comp5" bodies 17 removing the originals makes body 33 in component "Component''''"
copy_body "Body->Comp6" bodies 22 removing the originals makes body 34 in component "Component'''''"
copy_body "Body->Comp7" bodies 23 removing the originals makes body 35 in component "Component''''''"
copy_body "Body->Comp8" bodies 24 removing the originals makes body 36 in component "Component'''''''"
copy_body "Body->Comp9" bodies 25 removing the originals makes body 37 in component "Component''''''''"
copy_body "Body->Comp10" bodies 26 removing the originals makes body 38 in component "Component'''''''''"
copy_body "Body->Comp11" bodies 27 removing the originals makes body 39 in component "Component''''''''''"
copy_body "Body->Comp12" bodies 28 removing the originals makes body 40 in component "Component'''''''''''"
sketch "Sketch1 (2)" plane through (0, 0, 0) normal (0, 0, 1) x (1, 0, 0) in component "B&P SKETCH"
  line L0 (0, 0) -> (-200, 0)
  line L1 (-200, 0) -> (-200, 200)
  line L2 (-200, 200) -> (0, 200)
  line L3 (0, 200) -> (0, 0)
  dimension "d370" = 200
  dimension "d371" = 200
  constraint horizontal L0
  constraint vertical L1
  constraint horizontal L2
  constraint vertical L3
  constraint coincident L0.start L3.end
  measures "d370" distance of L0.start L0.end
  measures "d371" distance of L0.start L2.end
other "Arrange1"
sketch "Sketch1 (1)" plane through (0, 0, 0) normal (0, 0, 1) x (1, 0, 0) in component "B&P SKETCH"
  line L0 (0, 0) -> (200, 0)
  line L1 (200, 0) -> (200, 200)
  line L2 (200, 200) -> (0, 200)
  line L3 (0, 200) -> (0, 0)
  dimension "d413" = 200
  dimension "d414" = 200
  constraint horizontal L0
  constraint vertical L1
  constraint horizontal L2
  constraint vertical L3
  constraint coincident L0.start L3.end
  measures "d413" distance of L0.start L0.end
  measures "d414" distance of L0.start L2.end
other "Arrange2"
other "Arrange3"
component "Bakki" placed x (1, 0, 0) y (0, 1, 0) z (0, 0, 1) at (0, 0, 0)
component "Púsl" placed x (1, 0, 0) y (0, 1, 0) z (0, 0, 1) at (0, 0, 0)
component "CAM bakki" placed x (1, 0, 0) y (0, 1, 0) z (0, 0, 1) at (220.4262, -132.1769, 0)
component "CAM púsl" placed x (1, 0, 0) y (0, 1, 0) z (0, 0, 1) at (0, 0, 0)
component "B&P SKETCH" placed x (1, 0, 0) y (0, 1, 0) z (0, 0, 1) at (0, 0, 0)
component "Arrange1" placed x (1, 0, 0) y (0, 1, 0) z (0, 0, 1) at (0, 0, 0)
component "Arrange2" placed x (1, 0, 0) y (0, 1, 0) z (0, 0, 1) at (0, 0, 0)
component "Arrange3" placed x (1, 0, 0) y (0, 1, 0) z (0, 0, 1) at (0, 0, 0)
component "Component" placed x (1, 0, 0) y (0, 1, 0) z (0, 0, 1) at (0, 0, 0) in component "Bakki"
component "Component'" placed x (1, 0, 0) y (0, 1, 0) z (0, 0, 1) at (0, 0, 0) in component "Bakki"
component "Component''" placed x (1, 0, 0) y (0, 1, 0) z (0, 0, 1) at (0, 0, 0) in component "Bakki"
component "Component'''" placed x (1, 0, 0) y (0, 1, 0) z (0, 0, 1) at (0, 0, 0) in component "Bakki"
component "Component''''" placed x (1, 0, 0) y (0, 1, 0) z (0, 0, 1) at (0, 0, 0) in component "Bakki"
component "Component'''''''''''" placed x (1, 0, 0) y (0, 1, 0) z (0, 0, 1) at (0, 0, 0) in component "Púsl"
component "Component''''''''" placed x (1, 0, 0) y (0, 1, 0) z (0, 0, 1) at (0, 0, 0) in component "Púsl"
component "Component'''''''''" placed x (1, 0, 0) y (0, 1, 0) z (0, 0, 1) at (0, 0, 0) in component "Púsl"
component "Component'''''''" placed x (1, 0, 0) y (0, 1, 0) z (0, 0, 1) at (0, 0, 0) in component "Púsl"
component "Component''''''''''" placed x (1, 0, 0) y (0, 1, 0) z (0, 0, 1) at (0, 0, 0) in component "Púsl"
component "Component''''''" placed x (1, 0, 0) y (0, 1, 0) z (0, 0, 1) at (0, 0, 0) in component "Púsl"
component "Component'''''" placed x (1, 0, 0) y (0, 1, 0) z (0, 0, 1) at (0, 0, 0) in component "Púsl"
component "Component" placed x (1, 0, 0) y (0, 1, 0) z (0, 0, 1) at (-150, 0, 0) in component "CAM bakki"
component "Component'''" placed x (1, 0, 0) y (0, 0, 1) z (0, -1, 0) at (-319.8942, 51.9863, -83) in component "CAM bakki"
component "Component''''" placed x (0, 0, 1) y (0, 1, 0) z (-1, 0, 0) at (-157.6558, -0.9195, -118) in component "CAM bakki"
component "Component''" placed x (1, 0, 0) y (0, 0, -1) z (0, 1, 0) at (-320.529, 72.3598, 3) in component "CAM bakki"
component "Component'" placed x (0, 0, -1) y (0, 1, 0) z (1, 0, 0) at (-176.6225, -1.6023, 3) in component "CAM bakki"
component "Component'''''''''''" placed x (1, 0, 0) y (0, 1, 0) z (0, 0, 1) at (140, 0, 0) in component "CAM púsl"
component "Component'''''" placed x (1, 0, 0) y (0, 1, 0) z (0, 0, 1) at (140, 0, 0) in component "CAM púsl"
component "Component''''''''" placed x (1, 0, 0) y (0, 1, 0) z (0, 0, 1) at (140, 0, 0) in component "CAM púsl"
component "Component''''''''''" placed x (1, 0, 0) y (0, 1, 0) z (0, 0, 1) at (140, 0, 0) in component "CAM púsl"
component "Component''''''" placed x (1, 0, 0) y (0, 1, 0) z (0, 0, 1) at (140, 0, 0) in component "CAM púsl"
component "Component'''''''" placed x (1, 0, 0) y (0, 1, 0) z (0, 0, 1) at (140, 0, 0) in component "CAM púsl"
component "Component'''''''''" placed x (1, 0, 0) y (0, 1, 0) z (0, 0, 1) at (140, 0, 0) in component "CAM púsl"
component "Envelope1(Qty: 1)" placed x (1, 0, 0) y (0, 1, 0) z (0, 0, 1) at (-200, 0, 0) in component "Arrange1"
component "Component" placed x (1, 0, 0) y (0, 1, 0) z (0, 0, 1) at (6.35, 6.35, 0) in component "Envelope1(Qty: 1)"
component "Component'''" placed x (-1, 0, 0) y (0, 0, -1) z (0, -1, 0) at (124.55, 104.3, 86.4) in component "Envelope1(Qty: 1)"
component "Component''''" placed x (0, 0, 1) y (1, 0, 0) z (0, 1, 0) at (6.35, 128.2, -118.2) in component "Envelope1(Qty: 1)"
component "Component''" placed x (1, 0, 0) y (0, 0, -1) z (0, 1, 0) at (3.15, 114.65, 3.2) in component "Envelope1(Qty: 1)"
component "Component'" placed x (0, 0, 1) y (1, 0, 0) z (0, 1, 0) at (6.35, 141.75, 0) in component "Envelope1(Qty: 1)"
component "Envelope1(Qty: 1) (1)" placed x (1, 0, 0) y (0, 1, 0) z (0, 0, 1) at (0, 0, 0) in component "Arrange3"
component "Component'''''''''''" placed x (0, -1, 0) y (1, 0, 0) z (0, 0, 1) at (3.15, 150.9, -3.2) in component "Envelope1(Qty: 1) (1)"
component "Component'''''" placed x (0, 1, 0) y (-1, 0, 0) z (0, 0, 1) at (89.55, 3.15, -3.2) in component "Envelope1(Qty: 1) (1)"
component "Component''''''''" placed x (-1, 0, 0) y (0, -1, 0) z (0, 0, 1) at (104.55, 161.1454, -3.2) in component "Envelope1(Qty: 1) (1)"
component "Component''''''''''" placed x (-1, 0, 0) y (0, -1, 0) z (0, 0, 1) at (109.55, 104.7954, -3.2) in component "Envelope1(Qty: 1) (1)"
component "Component''''''" placed x (1, 0, 0) y (0, 1, 0) z (0, 0, 1) at (-16.85, 67.641, -3.2) in component "Envelope1(Qty: 1) (1)"
component "Component'''''''" placed x (-1, 0, 0) y (0, -1, 0) z (0, 0, 1) at (104.55, 225.391, -3.2) in component "Envelope1(Qty: 1) (1)"
component "Component'''''''''" placed x (1, 0, 0) y (0, 1, 0) z (0, 0, 1) at (-16.85, 40.85, -3.2) in component "Envelope1(Qty: 1) (1)"
equation "d1 = breidd + offset"
equation "d2 = lengd + offset"
equation "breidd = lengd + 7 / 3 * biti"
equation "þykkt = 3.2 mm"
equation "tönn = 10 mm"
equation "d6 = tönn"
equation "d7 = þykkt"
equation "d8 = offset"
equation "offset = 2 * þykkt"
equation "d12 = breidd - offset - tönn"
equation "d17 = lengd - þykkt + offset"
equation "d18 = þykkt"
equation "d19 = tönn"
equation "d20 = offset"
equation "d24 = lengd - offset - tönn"
equation "d27 = breidd + offset - þykkt"
equation "d29 = þykkt"
equation "hæð = 2 mm"
equation "lengd = 5 * biti + 1 / 3 * biti"
equation "d74 = þykkt"
equation "d75 = lengd + offset"
equation "d76 = -þykkt"
equation "d78 = þykkt"
equation "d79 = lengd + offset"
equation "d80 = hæð"
equation "d82 = þykkt"
equation "d83 = lengd + offset"
equation "d84 = hæð"
equation "d86 = breidd"
equation "d87 = þykkt"
equation "d88 = -þykkt"
equation "d90 = breidd"
equation "d91 = þykkt"
equation "d92 = hæð"
equation "d94 = breidd"
equation "d95 = þykkt"
equation "d96 = hæð"
equation "d98 = breidd"
equation "d99 = þykkt"
equation "d100 = -þykkt"
equation "d102 = hæð"
equation "d104 = breidd"
equation "d105 = þykkt"
equation "d106 = hæð"
equation "d108 = þykkt"
equation "d109 = lengd + offset"
equation "d110 = -þykkt"
equation "d112 = hæð"
equation "d114 = þykkt"
equation "d115 = lengd + offset"
equation "d116 = hæð"
equation "biti = 15 mm"
equation "rún = 2 mm"
equation "d178 = biti"
equation "d179 = 1 / 3 * biti"
equation "d180 = 1 / 3 * biti"
equation "d181 = 1 / 3 * biti"
equation "d182 = 3 * biti"
equation "d183 = 1 / 3 * biti"
equation "d185 = biti"
equation "d186 = 5 / 3 * biti"
equation "d187 = 1 / 3 * biti"
equation "d188 = rún"
equation "d189 = þykkt + 1 / 3 * biti"
equation "d190 = rún"
equation "d191 = rún"
equation "d192 = rún"
equation "d193 = rún"
equation "d194 = rún"
equation "d195 = rún"
equation "d196 = rún"
equation "d197 = rún"
equation "d198 = rún"
equation "d202 = 2 * biti"
equation "d203 = lengd"
equation "d204 = biti"
equation "d205 = þykkt + 4 / 3 * biti"
equation "d206 = þykkt + lengd"
equation "d208 = 1 / 4 * lengd - 1 / 6 * biti"
equation "d209 = 1 / 3 * biti"
equation "d210 = 1 / 3 * biti"
equation "d211 = 1 / 3 * biti"
equation "d212 = 3 / 4 * lengd - 1 / 6 * biti"
equation "d213 = 1 / 4 * lengd - 1 / 3 * biti"
equation "d214 = 1 / 3 * biti"
equation "d215 = 2 / 3 * biti"
equation "d216 = 1 / 3 * biti"
equation "d218 = 3 / 4 * lengd - 1 / 3 * biti"
equation "d219 = rún"
equation "d220 = rún"
equation "d221 = rún"
equation "d222 = rún"
equation "d223 = rún"
equation "d224 = rún"
equation "d225 = rún"
equation "d226 = rún"